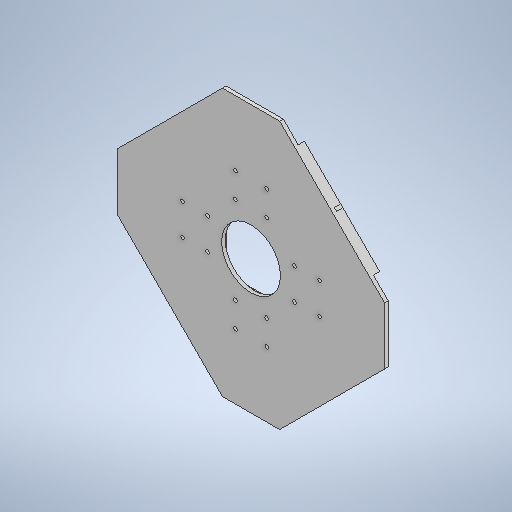
# Autodesk Inventor part: MainBase
Saved by Autodesk Inventor 2025.1 (Build 291241000, 241)
## iProperties
Created: 2025-05-09
Part Number: MainBase
Material: Generic
Document SubType Name: Modeling
Designer: User
Density: 1 g/cm^3
Appearance: Default
Author: User
## iProperties of the stored document MainBase_3DPrint.ipt
Created: 2025-05-09
Part Number: MainBase_3DPrint
Material: Generic
Document SubType Name: Modeling
Designer: User
Density: 1 g/cm^3
Appearance: Default
Author: User
Autodesk Inventor part; units mm, degrees
ref_plane "YZ Plane" through (0, 0, 0) normal (1, 0, 0) x (0, 1, 0)
ref_plane "XZ Plane" through (0, 0, 0) normal (0, 1, 0) x (-1, 0, 0)
ref_plane "XY Plane" through (0, 0, 0) normal (0, 0, 1) x (1, 0, 0)
sketch "Sketch1" plane through (0, 0, 0) normal (0, 0, 1) x (1, 0, 0)
  line L0 (0, 102.0898) -> (-155.5635, -53.4737) projected
  circle A0 centre (0, -53.4737) radius 15.2178 projected
  line L1 (0, -209.0372) -> (155.5635, -53.4737) projected
  line L2 (155.5635, -53.4737) -> (0, 102.0898) projected
  line L3 (0, 102.0898) -> (-155.5635, -53.4737) projected
  line L4 (-155.5635, -53.4737) -> (0, -209.0372) projected
  point P0 (0, 0)
extrude "Extrusion1" add sketch "Sketch1" along normal blind 3.5
sketch "Sketch3" plane through (0, 0, 0) normal (0, 0, -1) x (-1, 0, 0)
  circle A0 centre (-15, 12.25) radius 1.75 projected
  circle A1 centre (15, 12.25) radius 1.75 projected
  circle A2 centre (15, -11.75) radius 1.75 projected
  circle A3 centre (-15, -11.75) radius 1.75 projected
  circle A4 centre (-65.7237, -68.4737) radius 1.75 projected
  circle A5 centre (-41.7237, -68.4737) radius 1.75 projected
  circle A6 centre (-41.7237, -38.4737) radius 1.75 projected
  circle A7 centre (-65.7237, -38.4737) radius 1.75 projected
  circle A8 centre (-15, -95.1974) radius 1.75 projected
  circle A9 centre (-15, -119.1974) radius 1.75 projected
  circle A10 centre (15, -119.1974) radius 1.75 projected
  circle A11 centre (15, -95.1974) radius 1.75 projected
  circle A12 centre (41.7237, -68.4737) radius 1.75 projected
  circle A13 centre (65.7237, -68.4737) radius 1.75 projected
  circle A14 centre (41.7237, -38.4737) radius 1.75 projected
  circle A15 centre (65.7237, -38.4737) radius 1.75 projected
  point P0 (0, 0)
extrude "Extrusion2" cut sketch "Sketch3" against normal blind 3.5
sketch "Sketch4" plane through (0, 0, 0) normal (0, 0, -1) x (-1, 0, 0)
  line L0 (-76.2237, -73.4737) -> (-76.2237, -33.4737) projected
  line L1 (-36.2237, -33.4737) -> (-73.7237, -33.4737) projected
  line L2 (-33.7237, -70.9737) -> (-33.7237, -35.9737) projected
  line L3 (-73.7237, -73.4737) -> (-36.2237, -73.4737) projected
  line L4 (-73.7237, -73.4737) -> (-76.2237, -73.4737) projected
  line L5 (-76.2237, -33.4737) -> (-73.7237, -33.4737) projected
  arc A0 (-33.7237, -35.9737) -> (-36.2237, -33.4737) centre (-36.2237, -35.9737) ccw projected
  arc A1 (-36.2237, -73.4737) -> (-33.7237, -70.9737) centre (-36.2237, -70.9737) ccw projected
  line L6 (-20, -89.6974) -> (-20, -127.1974) projected
  arc A2 (-17.5, -87.1974) -> (-20, -89.6974) centre (-17.5, -89.6974) ccw projected
  line L7 (17.5, -87.1974) -> (-17.5, -87.1974) projected
  arc A3 (20, -89.6974) -> (17.5, -87.1974) centre (17.5, -89.6974) ccw projected
  line L8 (20, -124.1974) -> (20, -89.6974) projected
  line L9 (20, -129.6974) -> (-20, -129.6974) projected
  line L10 (-20, -129.6974) -> (-20, -127.1974) projected
  line L11 (20, -127.1974) -> (20, -129.6974) projected
  line L12 (20, -127.1974) -> (20, -89.6974) projected
  line L13 (36.2237, -73.4737) -> (73.7237, -73.4737) projected
  arc A4 (33.7237, -70.9737) -> (36.2237, -73.4737) centre (36.2237, -70.9737) ccw projected
  line L14 (33.7237, -35.9737) -> (33.7237, -70.9737) projected
  arc A5 (36.2237, -33.4737) -> (33.7237, -35.9737) centre (36.2237, -35.9737) ccw projected
  line L15 (73.7237, -33.4737) -> (36.2237, -33.4737) projected
  line L16 (73.7237, -33.4737) -> (76.2237, -33.4737) projected
  line L17 (76.2237, -33.4737) -> (76.2237, -73.4737) projected
  line L18 (76.2237, -73.4737) -> (73.7237, -73.4737) projected
  line L19 (20, -17.25) -> (20, 20.25) projected
  arc A6 (17.5, -19.75) -> (20, -17.25) centre (17.5, -17.25) ccw projected
  line L20 (-17.5, -19.75) -> (17.5, -19.75) projected
  arc A7 (-20, -17.25) -> (-17.5, -19.75) centre (-17.5, -17.25) ccw projected
  line L21 (-20, 20.25) -> (-20, -17.25) projected
  line L22 (-20, 20.25) -> (-20, 22.75) projected
  line L23 (20, 22.75) -> (20, 20.25) projected
  line L24 (-20, 22.75) -> (20, 22.75) projected
  arc A8 (-21, -17.25) -> (-17.5, -20.75) centre (-17.5, -17.25) ccw
  line L25 (-17.5, -20.75) -> (17.5, -20.75)
  arc A9 (17.5, -20.75) -> (21, -17.25) centre (17.5, -17.25) ccw
  line L26 (21, -17.25) -> (21, 20.25)
  line L27 (21, 20.25) -> (21, 23.75)
  line L28 (21, 23.75) -> (-21, 23.75)
  line L29 (-21, 23.75) -> (-21, 20.25)
  line L30 (-21, 20.25) -> (-21, -17.25)
  arc A10 (36.2237, -32.4737) -> (32.7237, -35.9737) centre (36.2237, -35.9737) ccw
  line L31 (32.7237, -35.9737) -> (32.7237, -70.9737)
  arc A11 (32.7237, -70.9737) -> (36.2237, -74.4737) centre (36.2237, -70.9737) ccw
  line L32 (36.2237, -74.4737) -> (73.7237, -74.4737)
  line L33 (73.7237, -74.4737) -> (77.2237, -74.4737)
  line L34 (77.2237, -74.4737) -> (77.2237, -32.4737)
  line L35 (77.2237, -32.4737) -> (73.7237, -32.4737)
  line L36 (73.7237, -32.4737) -> (36.2237, -32.4737)
  line L37 (-73.7237, -32.4737) -> (-36.2237, -32.4737)
  arc A12 (-32.7237, -35.9737) -> (-36.2237, -32.4737) centre (-36.2237, -35.9737) ccw
  line L38 (-32.7237, -35.9737) -> (-32.7237, -70.9737)
  arc A13 (-36.2237, -74.4737) -> (-32.7237, -70.9737) centre (-36.2237, -70.9737) ccw
  line L39 (-36.2237, -74.4737) -> (-73.7237, -74.4737)
  line L40 (-73.7237, -74.4737) -> (-77.2237, -74.4737)
  line L41 (-77.2237, -74.4737) -> (-77.2237, -32.4737)
  line L42 (-77.2237, -32.4737) -> (-73.7237, -32.4737)
  arc A14 (-17.5, -86.1974) -> (-21, -89.6974) centre (-17.5, -89.6974) ccw
  line L43 (-21, -89.6974) -> (-21, -127.1974)
  line L44 (-21, -127.1974) -> (-21, -130.6974)
  line L45 (-21, -130.6974) -> (21, -130.6974)
  line L46 (21, -130.6974) -> (21, -127.1974)
  line L47 (21, -127.1974) -> (21, -89.6974)
  arc A15 (21, -89.6974) -> (17.5, -86.1974) centre (17.5, -89.6974) ccw
  line L48 (17.5, -86.1974) -> (-17.5, -86.1974)
  point P0 (0, 0)
  dimension "d9" = 1
  dimension "d10" = 1
  dimension "d11" = 1
  dimension "d12" = 1
  constraints: 48 end point, 16 point on circle, 8 centre point, 28 other
  measures "d9" distance between parallel lines of L21 L30
  measures "d10" distance between parallel lines of L15 L36
  measures "d11" distance between parallel lines of L1 L37
  measures "d12" distance between parallel lines of L7 L48
extrude "Extrusion3" cut sketch "Sketch4" against normal blind 0.5 contours L0 L5 L1 A0 L2 A1 L3 L4 | A2 L7 A3 L8 L12 L11 L9 L10 L6 | A4 L14 A5 L15 L16 L17 L18 L13 | A6 L20 A7 L21 L22 L24 L23 L19 | L30 L29 L28 L27 L26 A9 L25 A8 | L36 L35 L34 L33 L32 A11 L31 A10 | L37 A12 L38 A13 L39 L40 L41 L42 | L48 A15 L47 L46 L45 L44 L43 A14
sketch "Sketch5" plane through (0, 0, 0) normal (0, 0, -1) x (-1, 0, 0)
  arc A0 (32.7237, -70.9737) -> (36.2237, -74.4737) centre (36.2237, -70.9737) ccw projected
  line L0 (32.7237, -70.9737) -> (32.7237, -35.9737) projected
  arc A1 (36.2237, -32.4737) -> (32.7237, -35.9737) centre (36.2237, -35.9737) ccw projected
  line L1 (36.2237, -32.4737) -> (77.2237, -32.4737) projected
  line L2 (77.2237, -32.4737) -> (77.2237, -74.4737) projected
  line L3 (77.2237, -74.4737) -> (36.2237, -74.4737) projected
  line L4 (21, -130.6974) -> (-21, -130.6974) projected
  line L5 (-21, -130.6974) -> (-21, -89.6974) projected
  arc A2 (-17.5, -86.1974) -> (-21, -89.6974) centre (-17.5, -89.6974) ccw projected
  line L6 (-17.5, -86.1974) -> (17.5, -86.1974) projected
  arc A3 (21, -89.6974) -> (17.5, -86.1974) centre (17.5, -89.6974) ccw projected
  line L7 (21, -89.6974) -> (21, -130.6974) projected
  arc A4 (17.5, -20.75) -> (21, -17.25) centre (17.5, -17.25) ccw projected
  line L8 (17.5, -20.75) -> (-17.5, -20.75) projected
  arc A5 (-21, -17.25) -> (-17.5, -20.75) centre (-17.5, -17.25) ccw projected
  line L9 (-21, -17.25) -> (-21, 23.75) projected
  line L10 (-21, 23.75) -> (21, 23.75) projected
  line L11 (21, 23.75) -> (21, -17.25) projected
  arc A6 (-32.7237, -35.9737) -> (-36.2237, -32.4737) centre (-36.2237, -35.9737) ccw projected
  line L12 (-32.7237, -35.9737) -> (-32.7237, -70.9737) projected
  arc A7 (-36.2237, -74.4737) -> (-32.7237, -70.9737) centre (-36.2237, -70.9737) ccw projected
  line L13 (-36.2237, -74.4737) -> (-77.2237, -74.4737) projected
  line L14 (-77.2237, -74.4737) -> (-77.2237, -32.4737) projected
  line L15 (-77.2237, -32.4737) -> (-36.2237, -32.4737) projected
  line L16 (0, 102.0898) -> (155.5635, -53.4737) projected
  line L17 (-155.5635, -53.4737) -> (0, 102.0898) projected
  line L18 (0, -209.0372) -> (-155.5635, -53.4737) projected
  line L19 (155.5635, -53.4737) -> (0, -209.0372) projected
  circle A8 centre (0, -53.4737) radius 15.2178 projected
  line L20 (-25.5, 28.25) -> (-25.5, -17.25)
  arc A9 (-25.5, -17.25) -> (-17.5, -25.25) centre (-17.5, -17.25) ccw
  line L21 (-17.5, -25.25) -> (17.5, -25.25)
  arc A10 (17.5, -25.25) -> (25.5, -17.25) centre (17.5, -17.25) ccw
  line L22 (25.5, -17.25) -> (25.5, 28.25)
  line L23 (25.5, 28.25) -> (-25.5, 28.25)
  arc A11 (-28.2237, -35.9737) -> (-36.2237, -27.9737) centre (-36.2237, -35.9737) ccw
  line L24 (-28.2237, -35.9737) -> (-28.2237, -70.9737)
  arc A12 (-36.2237, -78.9737) -> (-28.2237, -70.9737) centre (-36.2237, -70.9737) ccw
  line L25 (-36.2237, -78.9737) -> (-81.7237, -78.9737)
  line L26 (-81.7237, -78.9737) -> (-81.7237, -27.9737)
  line L27 (-81.7237, -27.9737) -> (-36.2237, -27.9737)
  line L28 (81.7237, -27.9737) -> (36.2237, -27.9737)
  arc A13 (36.2237, -27.9737) -> (28.2237, -35.9737) centre (36.2237, -35.9737) ccw
  line L29 (28.2237, -35.9737) -> (28.2237, -70.9737)
  arc A14 (28.2237, -70.9737) -> (36.2237, -78.9737) centre (36.2237, -70.9737) ccw
  line L30 (36.2237, -78.9737) -> (81.7237, -78.9737)
  line L31 (81.7237, -78.9737) -> (81.7237, -27.9737)
  line L32 (17.5, -81.6974) -> (-17.5, -81.6974)
  arc A15 (-17.5, -81.6974) -> (-25.5, -89.6974) centre (-17.5, -89.6974) ccw
  line L33 (-25.5, -89.6974) -> (-25.5, -135.1974)
  line L34 (-25.5, -135.1974) -> (25.5, -135.1974)
  line L35 (25.5, -135.1974) -> (25.5, -89.6974)
  arc A16 (25.5, -89.6974) -> (17.5, -81.6974) centre (17.5, -89.6974) ccw
  point P0 (0, 0)
  dimension "d15" = 4.5
  dimension "d16" = 4.5
  dimension "d17" = 4.5
  dimension "d18" = 4.5
  constraints: 32 end point, 16 point on circle, 8 centre point, 20 other
  measures "d15" distance between parallel lines of L9 L20
  measures "d16" distance between parallel lines of L15 L27
  measures "d17" distance between parallel lines of L1 L28
  measures "d18" radial gap between concentric circles of A3 A16
extrude "Extrusion4" add sketch "Sketch5" along normal blind 1 contours L23 L22 A10 L21 A9 L20 | L24 A12 L25 L26 L27 A11 | L31 L30 A14 L29 A13 L28 | A16 L35 L34 L33 A15 L32
sketch "Sketch6" plane through (0, 0, 0) normal (0, 0, -1) x (-1, 0, 0)
  line L0 (17.5, -81.6974) -> (-17.5, -81.6974) projected
  circle A0 centre (0, -53.4737) radius 15.2178 projected
  line L1 (-28.2237, -70.9737) -> (-28.2237, -35.9737) projected
  line L2 (-17.5, -25.25) -> (17.5, -25.25) projected
  circle A1 centre (0, -53.4737) radius 28.2237
  point P0 (0, 0)
  constraints: 1 centre point, 1 coincident
extrude "Extrusion5" cut sketch "Sketch6" against normal through all
sketch "Sketch7" plane through (0, 0, 0) normal (0, 0, -1) x (-1, 0, 0)
  line L0 (8, 74.65) -> (-8, 74.65) projected
  line L1 (128.1237, -61.4737) -> (128.1237, -45.4737) projected
  line L2 (-128.1237, -45.4737) -> (-128.1237, -61.4737) projected
  line L3 (0, 102.0898) -> (155.5635, -53.4737) projected
  line L4 (-155.5635, -53.4737) -> (0, 102.0898) projected
  line L5 (0, -209.0372) -> (-155.5635, -53.4737) projected
  line L6 (155.5635, -53.4737) -> (0, -209.0372) projected
  arc A0 (-36.2237, -78.9737) -> (-28.2237, -70.9737) centre (-36.2237, -70.9737) ccw projected
  line L7 (-36.2237, -78.9737) -> (-81.7237, -78.9737) projected
  line L8 (-81.7237, -78.9737) -> (-81.7237, -27.9737) projected
  line L9 (-81.7237, -27.9737) -> (-36.2237, -27.9737) projected
  arc A1 (-28.2237, -35.9737) -> (-36.2237, -27.9737) centre (-36.2237, -35.9737) ccw projected
  line L10 (-28.2237, -35.9737) -> (-28.2237, -53.4737) projected
  arc A2 (0, -25.25) -> (-28.2237, -53.4737) centre (0, -53.4737) ccw projected
  line L11 (0, -25.25) -> (-17.5, -25.25) projected
  arc A3 (-25.5, -17.25) -> (-17.5, -25.25) centre (-17.5, -17.25) ccw projected
  line L12 (-25.5, -17.25) -> (-25.5, 28.25) projected
  line L13 (-25.5, 28.25) -> (25.5, 28.25) projected
  line L14 (25.5, 28.25) -> (25.5, -17.25) projected
  arc A4 (17.5, -25.25) -> (25.5, -17.25) centre (17.5, -17.25) ccw projected
  line L15 (17.5, -25.25) -> (0, -25.25) projected
  arc A5 (28.2237, -53.4737) -> (0, -25.25) centre (0, -53.4737) ccw projected
  line L16 (28.2237, -53.4737) -> (28.2237, -35.9737) projected
  arc A6 (36.2237, -27.9737) -> (28.2237, -35.9737) centre (36.2237, -35.9737) ccw projected
  line L17 (36.2237, -27.9737) -> (81.7237, -27.9737) projected
  line L18 (81.7237, -27.9737) -> (81.7237, -78.9737) projected
  line L19 (81.7237, -78.9737) -> (36.2237, -78.9737) projected
  arc A7 (28.2237, -70.9737) -> (36.2237, -78.9737) centre (36.2237, -70.9737) ccw projected
  line L20 (28.2237, -70.9737) -> (28.2237, -53.4737) projected
  arc A8 (0, -81.6974) -> (28.2237, -53.4737) centre (0, -53.4737) ccw projected
  line L21 (0, -81.6974) -> (17.5, -81.6974) projected
  arc A9 (25.5, -89.6974) -> (17.5, -81.6974) centre (17.5, -89.6974) ccw projected
  line L22 (25.5, -89.6974) -> (25.5, -135.1974) projected
  line L23 (25.5, -135.1974) -> (-25.5, -135.1974) projected
  line L24 (-25.5, -135.1974) -> (-25.5, -89.6974) projected
  arc A10 (-17.5, -81.6974) -> (-25.5, -89.6974) centre (-17.5, -89.6974) ccw projected
  line L25 (-17.5, -81.6974) -> (0, -81.6974) projected
  arc A11 (-28.2237, -53.4737) -> (0, -81.6974) centre (0, -53.4737) ccw projected
  line L26 (-28.2237, -53.4737) -> (-28.2237, -70.9737) projected
  line L27 (-8, -181.5974) -> (8, -181.5974) projected
  line L28 (-27.4398, -181.5974) -> (27.4398, -181.5974)
  line L29 (128.1237, -80.9135) -> (128.1237, -26.0339)
  line L30 (8, 74.65) -> (27.4398, 74.65)
  line L31 (27.4398, 74.65) -> (-27.4398, 74.65)
  line L32 (-128.1237, -26.0339) -> (-128.1237, -80.9135)
  line L33 (-128.1237, -26.0339) -> (-155.5635, -53.4737)
  line L34 (-128.1237, -80.9135) -> (-155.5635, -53.4737)
  line L35 (-27.4398, -181.5974) -> (0, -209.0372)
  line L36 (27.4398, -181.5974) -> (0, -209.0372)
  line L37 (128.1237, -80.9135) -> (155.5635, -53.4737)
  line L38 (128.1237, -26.0339) -> (155.5635, -53.4737)
  line L39 (-27.4398, 74.65) -> (0, 102.0898)
  line L40 (0, 102.0898) -> (27.4398, 74.65)
  point P0 (0, 0)
  constraints: 26 end point, 10 point on line, 5 collinear, 3 perpendicular, 1 horizontal
extrude "Extrusion6" cut sketch "Sketch7" against normal blind 10 contours L0 L31 L4 L3 L30 | L3 L6 L29 L1 | L32 L2 L5 L4 | L6 L5 L28 L27
sketch "Sketch8" plane through (0, 0, 0) normal (0, 0, -1) x (-1, 0, 0)
  arc A0 (36.2237, -27.9737) -> (28.2237, -35.9737) centre (36.2237, -35.9737) ccw projected
  arc A1 (17.5, -25.25) -> (25.5, -17.25) centre (17.5, -17.25) ccw projected
  line L0 (30.5668, -30.3168) -> (23.1569, -22.9069)
  line L1 (26.8618, -26.6118) -> (77.0385, 25.0513)
  line L2 (27.4398, 74.65) -> (128.1237, -26.0339) projected
  line L3 (24.7403, -24.4903) -> (74.8864, 27.1415)
  line L4 (29.0139, -28.702) -> (79.1905, 22.9612)
  line L5 (79.1905, 22.9612) -> (74.8864, 27.1415)
  circle A2 centre (0, -53.4737) radius 15.2178 projected
  line L6 (-24.7717, -24.4598) -> (-76.4349, 25.7168)
  line L7 (-28.9834, -28.7334) -> (-80.6152, 21.4127)
  line L8 (-23.1569, -22.9069) -> (-30.5668, -30.3168)
  line L9 (-76.4349, 25.7168) -> (-80.6152, 21.4127)
  line L10 (-29.0139, -78.2454) -> (-79.1905, -129.9086)
  line L11 (-24.7403, -82.4571) -> (-74.8864, -134.0889)
  line L12 (-30.5668, -76.6305) -> (-23.1569, -84.0405)
  line L13 (-79.1905, -129.9086) -> (-74.8864, -134.0889)
  line L14 (24.7717, -82.4876) -> (76.4349, -132.6642)
  line L15 (28.9834, -78.214) -> (80.6152, -128.3601)
  line L16 (23.1569, -84.0405) -> (30.5668, -76.6305)
  line L17 (76.4349, -132.6642) -> (80.6152, -128.3601)
  line L18 (24.7403, -82.4571) -> (28.9834, -78.214)
  line L19 (29.0139, -28.702) -> (24.7403, -24.4903)
  line L20 (-28.9834, -28.7334) -> (-24.7717, -24.4598)
  line L21 (-29.0139, -78.2454) -> (-24.7403, -82.4571)
  line L22 (24.7717, -82.4876) -> (28.9834, -78.214)
  point P0 (0, 0)
  point P1 (-26.8618, -26.6118)
  point P2 (-26.8618, -80.3355)
  point P3 (26.8618, -80.3355)
  point P4 (79.16, 22.9298)
  point P5 (77.0385, 25.0513)
  dimension "d25" = 3
  dimension "d26" = 3
  dimension "d29" = 360
  constraints: 44 end point, 5 point on line, 3 perpendicular, 2 parallel, 2 point on circle, 1 collinear, 1 midpoint, 45 other
  measures "d25" distance between parallel lines of L1 L3
  measures "d26" distance between parallel lines of L1 L4
extrude "Extrusion7" add sketch "Sketch8" along normal blind 6 contours L3 L5 L1 L19 | L1 L2 L4 L19 | L20 L7 L9 L6 | L21 L11 L13 L10 | L22 L15 L17 L14
sketch "Sketch9" plane through (0, 0, 0) normal (0, 0, -1) x (-1, 0, 0)
  line L0 (82.7237, -56.4737) -> (81.7237, -56.4737)
  line L1 (94.2237, -50.4737) -> (81.7237, -50.4737)
  line L2 (128.1237, -80.9135) -> (128.1237, -26.0339) projected
  line L3 (100.9237, -54.9981) -> (100.9237, -48.2804) projected
  line L4 (81.7237, -27.9737) -> (81.7237, -78.9737) projected
  line L5 (81.7237, -50.4737) -> (94.8499, -50.4737)
  line L6 (100.8499, -50.4737) -> (100.8499, -56.4737)
  line L7 (94.8499, -56.4737) -> (81.7237, -56.4737)
  line L8 (81.7237, -56.4737) -> (81.7237, -50.4737)
  line L9 (114.3737, -24.8621) -> (104.3737, -24.8621) projected
  line L10 (104.3737, -82.233) -> (114.3737, -82.233) projected
  line L11 (94.8499, -50.4737) -> (94.8499, -24.7883)
  line L12 (100.8499, -24.7883) -> (100.8499, -50.4737)
  line L13 (94.8499, -56.4737) -> (94.8499, -82.1591)
  line L14 (100.8499, -82.1591) -> (100.8499, -56.4737)
  line L15 (81.7237, -56.4737) -> (81.7237, -50.4737)
  line L16 (100.8499, -24.7883) -> (113.864, -11.7742)
  line L17 (79.16, 22.9298) -> (128.1237, -26.0339) projected
  line L18 (94.8499, -24.7883) -> (110.864, -8.7742)
  line L19 (113.864, -11.7742) -> (110.864, -8.7742)
  line L20 (100.8499, -82.1591) -> (113.864, -95.1732)
  line L21 (94.8499, -82.1591) -> (110.864, -98.1732)
  line L22 (128.1237, -80.9135) -> (27.4398, -181.5974) projected
  line L23 (94.8499, -82.1591) -> (117.4972, -82.1591) construction
  line L24 (110.864, -98.1732) -> (113.864, -95.1732)
  line L25 (28.6854, 41.3762) -> (28.6854, 64.0235) construction
  line L26 (28.6854, 47.3762) -> (41.6995, 60.3903)
  line L27 (28.6854, 41.3762) -> (44.6995, 57.3903)
  line L28 (44.6995, 57.3903) -> (41.6995, 60.3903)
  line L29 (-28.6854, 47.3762) -> (-41.6995, 60.3903)
  line L30 (-28.6854, 41.3762) -> (-44.6995, 57.3903)
  line L31 (-41.6995, 60.3903) -> (-44.6995, 57.3903)
  line L32 (3, 29.25) -> (3, 28.25)
  line L33 (-3, 40.75) -> (-3, 28.25)
  line L34 (3, 41.3762) -> (28.6854, 41.3762)
  line L35 (28.6854, 47.3762) -> (3, 47.3762)
  line L36 (3, 41.3762) -> (3, 28.25)
  line L37 (-3, 28.25) -> (-3, 41.3762)
  line L38 (-3, 47.3762) -> (3, 47.3762)
  line L39 (3, 28.25) -> (-3, 28.25)
  line L40 (3, 28.25) -> (-3, 28.25)
  line L41 (-3, 41.3762) -> (-28.6854, 41.3762)
  line L42 (-28.6854, 47.3762) -> (-3, 47.3762)
  line L43 (-94.8499, -24.7883) -> (-117.4972, -24.7883) construction
  line L44 (-100.8499, -24.7883) -> (-113.864, -11.7742)
  line L45 (-94.8499, -24.7883) -> (-110.864, -8.7742)
  line L46 (-110.864, -8.7742) -> (-113.864, -11.7742)
  line L47 (-100.8499, -82.1591) -> (-113.864, -95.1732)
  line L48 (-94.8499, -82.1591) -> (-110.864, -98.1732)
  line L49 (-113.864, -95.1732) -> (-110.864, -98.1732)
  line L50 (-82.7237, -50.4737) -> (-81.7237, -50.4737)
  line L51 (-94.2237, -56.4737) -> (-81.7237, -56.4737)
  line L52 (-94.8499, -50.4737) -> (-94.8499, -24.7883)
  line L53 (-100.8499, -24.7883) -> (-100.8499, -50.4737)
  line L54 (-94.8499, -50.4737) -> (-81.7237, -50.4737)
  line L55 (-81.7237, -56.4737) -> (-94.8499, -56.4737)
  line L56 (-100.8499, -56.4737) -> (-100.8499, -50.4737)
  line L57 (-81.7237, -50.4737) -> (-81.7237, -56.4737)
  line L58 (-81.7237, -50.4737) -> (-81.7237, -56.4737)
  line L59 (-94.8499, -56.4737) -> (-94.8499, -82.1591)
  line L60 (-100.8499, -82.1591) -> (-100.8499, -56.4737)
  line L61 (-28.6854, -148.3236) -> (-28.6854, -170.9709) construction
  line L62 (-28.6854, -154.3236) -> (-41.6995, -167.3377)
  line L63 (-28.6854, -148.3236) -> (-44.6995, -164.3377)
  line L64 (-44.6995, -164.3377) -> (-41.6995, -167.3377)
  line L65 (28.6854, -154.3236) -> (41.6995, -167.3377)
  line L66 (28.6854, -148.3236) -> (44.6995, -164.3377)
  line L67 (41.6995, -167.3377) -> (44.6995, -164.3377)
  line L68 (-3, -136.1974) -> (-3, -135.1974)
  line L69 (3, -147.6974) -> (3, -135.1974)
  line L70 (-3, -148.3236) -> (-28.6854, -148.3236)
  line L71 (-28.6854, -154.3236) -> (-3, -154.3236)
  line L72 (-3, -148.3236) -> (-3, -135.1974)
  line L73 (3, -135.1974) -> (3, -148.3236)
  line L74 (3, -154.3236) -> (-3, -154.3236)
  line L75 (-3, -135.1974) -> (3, -135.1974)
  line L76 (-3, -135.1974) -> (3, -135.1974)
  line L77 (3, -148.3236) -> (28.6854, -148.3236)
  line L78 (28.6854, -154.3236) -> (3, -154.3236)
  point P0 (0, 0)
  point P1 (0, -53.4737)
  dimension "d34" = 45
  dimension "d37" = 360
  constraints: 144 end point, 8 point on line, 6 parallel, 4 horizontal, 3 perpendicular, 1 collinear, 1 equal length, 145 other
  measures "d34" angle of L21 L23
extrude "Extrusion8" add sketch "Sketch9" along normal blind 6 contours L0 L4 L1 L5 L11 L18 L17 L16 L12 L6 L14 L20 L22 L21 L13 L7 | L22 L65 L78 L74 L71 L62 L64 L63 L70 L72 L68 L75 L69 L73 L77 L66 | L26 L28 L27 L34 L36 L32 L39 L33 L37 L41 L30 L31 L29 L42 L38 L35 | L44 L46 L45 L52 L54 L50 L57 L51 L55 L59 L48 L49 L47 L60 L56 L53
sketch "Sketch10" plane through (0, 0, 0) normal (0, 0, -1) x (-1, 0, 0)
  line L0 (-110.864, -98.1732) -> (-94.8499, -82.1591) projected
  line L1 (-28.6854, -148.3236) -> (-44.6995, -164.3377) projected
  line L2 (-44.6995, -164.3377) -> (-77.0385, -131.9987) projected
  line L3 (0, -209.0372) -> (-155.5635, -53.4737) projected
  line L4 (-110.864, -98.1732) -> (-44.6995, -164.3377)
  line L5 (-44.6995, -164.3377) -> (-40.4569, -160.095)
  line L6 (-40.4569, -160.095) -> (-106.6213, -93.9306)
  line L7 (-106.6213, -93.9306) -> (-110.864, -98.1732)
  line L8 (44.6995, -164.3377) -> (110.864, -98.1732)
  line L9 (110.864, -98.1732) -> (106.6213, -93.9306)
  line L10 (106.6213, -93.9306) -> (40.4569, -160.095)
  line L11 (40.4569, -160.095) -> (44.6995, -164.3377)
  line L12 (110.864, -8.7742) -> (44.6995, 57.3903)
  line L13 (44.6995, 57.3903) -> (40.4569, 53.1476)
  line L14 (40.4569, 53.1476) -> (106.6213, -13.0168)
  line L15 (106.6213, -13.0168) -> (110.864, -8.7742)
  line L16 (-44.6995, 57.3903) -> (-110.864, -8.7742)
  line L17 (-110.864, -8.7742) -> (-106.6213, -13.0168)
  line L18 (-106.6213, -13.0168) -> (-40.4569, 53.1476)
  line L19 (-40.4569, 53.1476) -> (-44.6995, 57.3903)
  point P0 (0, 0)
  point P1 (0, -53.4737)
  dimension "d41" = 6
  dimension "d44" = 360
  constraints: 32 end point, 2 parallel, 2 perpendicular, 33 other
  measures "d41" distance of L5.end L1.end
extrude "Extrusion9" add sketch "Sketch10" along normal blind 6
chamfer "Chamfer1" distance 4 angle 45 4 edges at (100.8499, -53.4737, -6) (0, -154.3236, -6) (-100.8499, -53.4737, -6) (0, 47.3762, -6)
chamfer "Chamfer2" distance 3 angle 45 8 edges at (26.8771, -80.3512, -6) (26.8776, -26.5966, -6) (-26.8771, -26.5961, -6) (-26.8776, -80.3508, -6) (81.7237, -53.4737, -6) (0, -135.1974, -6) (-81.7237, -53.4737, -6) (0, 28.25, -6)
body "Solid1"
